Autodesk Inventor part; units mm, degrees
(part 2 of 2)
  line L254 (8.0901, 0.2026) -> (9.8203, 0.2026)
  line L255 (9.8203, 0.2026) -> (9.8203, -0.2399)
  spline S290 degree 2 poles (9.5423, 2.2873) (9.582, 2.2334) (9.7239, 2.0519) (9.7664, 1.9668) knots 0 0 0 1 2 2 2
  spline S291 degree 2 poles (9.7664, 1.9668) (9.8288, 1.8505) (9.894, 1.6321) (9.894, 1.4335) knots 0 0 0 1 2 2 2
  spline S292 degree 2 poles (9.894, 1.4335) (9.894, 1.2719) (9.7721, 0.9797) (9.6615, 0.8691) knots 0 0 0 1 2 2 2
  spline S293 degree 2 poles (9.6615, 0.8691) (9.5537, 0.7642) (9.236, 0.6365) (9.0602, 0.6365) knots 0 0 0 1 2 2 2
  spline S294 degree 2 poles (9.0602, 0.6365) (8.7879, 0.6365) (8.4021, 0.8663) (8.2915, 1.1159) knots 0 0 0 1 2 2 2
  spline S295 degree 2 poles (8.2915, 1.1159) (8.1894, 1.3371) (8.1128, 1.9384) (8.093, 2.2873) knots 0 0 0 1 2 2 2
  line L256 (8.093, 2.2873) -> (8.0079, 2.2873)
  spline S296 degree 2 poles (8.0079, 2.2873) (7.8547, 2.2873) (7.6647, 2.1937) (7.6108, 2.1086) knots 0 0 0 1 2 2 2
  spline S297 degree 2 poles (7.6108, 2.1086) (7.5569, 2.0235) (7.5229, 1.7796) (7.5229, 1.6491) knots 0 0 0 1 2 2 2
  spline S298 degree 2 poles (7.5229, 1.6491) (7.5229, 1.4959) (7.6136, 1.0818) (7.7016, 0.8748) knots 0 0 0 1 2 2 2
  line L257 (7.7016, 0.8748) -> (7.7016, 0.8493)
  line L258 (7.7016, 0.8493) -> (7.2506, 0.8493)
  spline S299 degree 2 poles (7.2506, 0.8493) (7.2166, 0.9712) (7.1315, 1.4279) (7.1315, 1.6519) knots 0 0 0 1 2 2 2
  spline S300 degree 2 poles (7.1315, 1.6519) (7.1315, 1.9242) (7.2166, 2.2958) (7.3272, 2.4433) knots 0 0 0 1 2 2 2
  spline S301 degree 2 poles (7.3272, 2.4433) (7.435, 2.5879) (7.7781, 2.7297) (8.0249, 2.7297) knots 0 0 0 1 2 2 2
  line L259 (8.0249, 2.7297) -> (9.8203, 2.7297)
  line L260 (9.8203, 2.7297) -> (9.8203, 2.2873)
  line L261 (9.8203, 2.2873) -> (9.5423, 2.2873)
  line L262 (9.1736, 2.2873) -> (8.4447, 2.2873)
  spline S302 degree 2 poles (8.4447, 2.2873) (8.4589, 2.1284) (8.5071, 1.6491) (8.5525, 1.4988) knots 0 0 0 1 2 2 2
  spline S303 degree 2 poles (8.5525, 1.4988) (8.6063, 1.3229) (8.8304, 1.0932) (9.029, 1.0932) knots 0 0 0 1 2 2 2
  spline S304 degree 2 poles (9.029, 1.0932) (9.2559, 1.0932) (9.4856, 1.3484) (9.4856, 1.5924) knots 0 0 0 1 2 2 2
  spline S305 degree 2 poles (9.4856, 1.5924) (9.4856, 1.7994) (9.3069, 2.1398) (9.1736, 2.2873) knots 0 0 0 1 2 2 2
  line L263 (9.8203, 5.3703) -> (9.8203, 4.9279)
  line L264 (9.8203, 4.9279) -> (9.5537, 4.9279)
  spline S306 degree 2 poles (9.5537, 4.9279) (9.6388, 4.8258) (9.7522, 4.6754) (9.8004, 4.5733) knots 0 0 0 1 2 2 2
  spline S307 degree 2 poles (9.8004, 4.5733) (9.8458, 4.4797) (9.894, 4.2784) (9.894, 4.145) knots 0 0 0 1 2 2 2
  spline S308 degree 2 poles (9.894, 4.145) (9.894, 3.9295) (9.7153, 3.5664) (9.5423, 3.4388) knots 0 0 0 1 2 2 2
  spline S309 degree 2 poles (9.5423, 3.4388) (9.3693, 3.3112) (8.8588, 3.1694) (8.5269, 3.1694) knots 0 0 0 1 2 2 2
  spline S310 degree 2 poles (8.5269, 3.1694) (8.1809, 3.1694) (7.676, 3.348) (7.486, 3.504) knots 0 0 0 1 2 2 2
  spline S311 degree 2 poles (7.486, 3.504) (7.3158, 3.6487) (7.1201, 4.0543) (7.1201, 4.2784) knots 0 0 0 1 2 2 2
  spline S312 degree 2 poles (7.1201, 4.2784) (7.1201, 4.4741) (7.208, 4.7662) (7.2988, 4.9279) knots 0 0 0 1 2 2 2
  line L265 (7.2988, 4.9279) -> (6.1643, 4.9279)
  line L266 (6.1643, 4.9279) -> (6.1643, 5.3703)
  line L267 (6.1643, 5.3703) -> (9.8203, 5.3703)
  line L268 (9.1821, 4.9279) -> (7.6647, 4.9279)
  spline S313 degree 2 poles (7.6647, 4.9279) (7.5853, 4.7634) (7.5257, 4.5024) (7.5257, 4.3521) knots 0 0 0 1 2 2 2
  spline S314 degree 2 poles (7.5257, 4.3521) (7.5257, 4.0117) (8.0362, 3.626) (8.5184, 3.626) knots 0 0 0 1 2 2 2
  spline S315 degree 2 poles (8.5184, 3.626) (8.9836, 3.626) (9.4743, 3.921) (9.4743, 4.2472) knots 0 0 0 1 2 2 2
  spline S316 degree 2 poles (9.4743, 4.2472) (9.4743, 4.4202) (9.3154, 4.7719) (9.1821, 4.9279) knots 0 0 0 1 2 2 2
  spline S317 degree 2 poles (9.8827, 8.5243) (9.8827, 8.1442) (9.7239, 7.611) (9.6104, 7.3756) knots 0 0 0 1 2 2 2
  line L269 (9.6104, 7.3756) -> (9.0261, 7.3756)
  line L270 (9.0261, 7.3756) -> (9.0261, 7.4096)
  spline S318 degree 2 poles (9.0261, 7.4096) (9.2417, 7.6394) (9.4799, 8.2208) (9.4799, 8.4903) knots 0 0 0 1 2 2 2
  spline S319 degree 2 poles (9.4799, 8.4903) (9.4799, 8.876) (9.1594, 9.2702) (8.8956, 9.2702) knots 0 0 0 1 2 2 2
  spline S320 degree 2 poles (8.8956, 9.2702) (8.6858, 9.2702) (8.4248, 9.0632) (8.3596, 8.8391) knots 0 0 0 1 2 2 2
  spline S321 degree 2 poles (8.3596, 8.8391) (8.3142, 8.6775) (8.2518, 8.408) (8.2008, 8.2066) knots 0 0 0 1 2 2 2
  spline S322 degree 2 poles (8.2008, 8.2066) (8.1525, 8.0251) (8.0079, 7.7386) (7.8916, 7.628) knots 0 0 0 1 2 2 2
  spline S323 degree 2 poles (7.8916, 7.628) (7.7753, 7.5202) (7.4633, 7.4011) (7.2591, 7.4011) knots 0 0 0 1 2 2 2
  spline S324 degree 2 poles (7.2591, 7.4011) (6.8337, 7.4011) (6.2579, 8.0648) (6.2579, 8.5782) knots 0 0 0 1 2 2 2
  spline S325 degree 2 poles (6.2579, 8.5782) (6.2579, 8.8732) (6.3742, 9.395) (6.4848, 9.6191) knots 0 0 0 1 2 2 2
  line L271 (6.4848, 9.6191) -> (7.0407, 9.6191)
  line L272 (7.0407, 9.6191) -> (7.0407, 9.5851)
  spline S326 degree 2 poles (7.0407, 9.5851) (6.8875, 9.4177) (6.6606, 8.8959) (6.6606, 8.6094) knots 0 0 0 1 2 2 2
  spline S327 degree 2 poles (6.6606, 8.6094) (6.6606, 8.286) (6.9641, 7.8861) (7.2109, 7.8861) knots 0 0 0 1 2 2 2
  spline S328 degree 2 poles (7.2109, 7.8861) (7.4321, 7.8861) (7.6959, 8.1215) (7.7555, 8.3428) knots 0 0 0 1 2 2 2
  spline S329 degree 2 poles (7.7555, 8.3428) (7.7952, 8.4903) (7.8973, 8.9185) (7.9398, 9.0604) knots 0 0 0 1 2 2 2
  spline S330 degree 2 poles (7.9398, 9.0604) (8.0504, 9.4206) (8.4957, 9.7553) (8.8219, 9.7553) knots 0 0 0 1 2 2 2
  spline S331 degree 2 poles (8.8219, 9.7553) (9.029, 9.7553) (9.426, 9.5879) (9.565, 9.4376) knots 0 0 0 1 2 2 2
  spline S332 degree 2 poles (9.565, 9.4376) (9.7182, 9.2702) (9.8827, 8.8448) (9.8827, 8.5243) knots 0 0 0 1 2 2 2
  spline S333 degree 2 poles (9.5423, 11.6584) (9.582, 11.6045) (9.7239, 11.423) (9.7664, 11.3379) knots 0 0 0 1 2 2 2
  spline S334 degree 2 poles (9.7664, 11.3379) (9.8288, 11.2216) (9.894, 11.0032) (9.894, 10.8047) knots 0 0 0 1 2 2 2
  spline S335 degree 2 poles (9.894, 10.8047) (9.894, 10.643) (9.7721, 10.3509) (9.6615, 10.2403) knots 0 0 0 1 2 2 2
  spline S336 degree 2 poles (9.6615, 10.2403) (9.5537, 10.1353) (9.236, 10.0077) (9.0602, 10.0077) knots 0 0 0 1 2 2 2
  spline S337 degree 2 poles (9.0602, 10.0077) (8.7879, 10.0077) (8.4021, 10.2374) (8.2915, 10.487) knots 0 0 0 1 2 2 2
  spline S338 degree 2 poles (8.2915, 10.487) (8.1894, 10.7083) (8.1128, 11.3096) (8.093, 11.6584) knots 0 0 0 1 2 2 2
  line L273 (8.093, 11.6584) -> (8.0079, 11.6584)
  spline S339 degree 2 poles (8.0079, 11.6584) (7.8547, 11.6584) (7.6647, 11.5648) (7.6108, 11.4797) knots 0 0 0 1 2 2 2
  spline S340 degree 2 poles (7.6108, 11.4797) (7.5569, 11.3946) (7.5229, 11.1507) (7.5229, 11.0202) knots 0 0 0 1 2 2 2
  spline S341 degree 2 poles (7.5229, 11.0202) (7.5229, 10.8671) (7.6136, 10.453) (7.7016, 10.2459) knots 0 0 0 1 2 2 2
  line L274 (7.7016, 10.2459) -> (7.7016, 10.2204)
  line L275 (7.7016, 10.2204) -> (7.2506, 10.2204)
  spline S342 degree 2 poles (7.2506, 10.2204) (7.2166, 10.3424) (7.1315, 10.799) (7.1315, 11.0231) knots 0 0 0 1 2 2 2
  spline S343 degree 2 poles (7.1315, 11.0231) (7.1315, 11.2954) (7.2166, 11.6669) (7.3272, 11.8144) knots 0 0 0 1 2 2 2
  spline S344 degree 2 poles (7.3272, 11.8144) (7.435, 11.9591) (7.7781, 12.1009) (8.0249, 12.1009) knots 0 0 0 1 2 2 2
  line L276 (8.0249, 12.1009) -> (9.8203, 12.1009)
  line L277 (9.8203, 12.1009) -> (9.8203, 11.6584)
  line L278 (9.8203, 11.6584) -> (9.5423, 11.6584)
  line L279 (9.1736, 11.6584) -> (8.4447, 11.6584)
  spline S345 degree 2 poles (8.4447, 11.6584) (8.4589, 11.4996) (8.5071, 11.0202) (8.5525, 10.8699) knots 0 0 0 1 2 2 2
  spline S346 degree 2 poles (8.5525, 10.8699) (8.6063, 10.6941) (8.8304, 10.4643) (9.029, 10.4643) knots 0 0 0 1 2 2 2
  spline S347 degree 2 poles (9.029, 10.4643) (9.2559, 10.4643) (9.4856, 10.7196) (9.4856, 10.9635) knots 0 0 0 1 2 2 2
  spline S348 degree 2 poles (9.4856, 10.9635) (9.4856, 11.1706) (9.3069, 11.5109) (9.1736, 11.6584) knots 0 0 0 1 2 2 2
  line L280 (9.8203, 13.173) -> (9.8203, 12.7305)
  line L281 (9.8203, 12.7305) -> (7.1939, 12.7305)
  line L282 (7.1939, 12.7305) -> (7.1939, 13.173)
  line L283 (7.1939, 13.173) -> (9.8203, 13.173)
  line L284 (6.7571, 13.2042) -> (6.7571, 12.7022)
  line L285 (6.7571, 12.7022) -> (6.2976, 12.7022)
  line L286 (6.2976, 12.7022) -> (6.2976, 13.2042)
  line L287 (6.2976, 13.2042) -> (6.7571, 13.2042)
  line L288 (6.5897, 15.2038) -> (6.5897, 15.1811)
  spline S349 degree 2 poles (6.5897, 15.1811) (6.567, 15.1215) (6.5273, 14.9003) (6.5273, 14.8124) knots 0 0 0 1 2 2 2
  spline S350 degree 2 poles (6.5273, 14.8124) (6.5273, 14.5344) (6.7769, 14.2962) (7.1059, 14.2962) knots 0 0 0 1 2 2 2
  line L289 (7.1059, 14.2962) -> (7.1939, 14.2962)
  line L290 (7.1939, 14.2962) -> (7.1939, 15.0279)
  line L291 (7.1939, 15.0279) -> (7.5598, 15.0279)
  line L292 (7.5598, 15.0279) -> (7.5598, 14.3104)
  line L293 (7.5598, 14.3104) -> (9.8203, 14.3104)
  line L294 (9.8203, 14.3104) -> (9.8203, 13.8679)
  line L295 (9.8203, 13.8679) -> (7.5598, 13.8679)
  line L296 (7.5598, 13.8679) -> (7.5598, 13.5701)
  line L297 (7.5598, 13.5701) -> (7.1939, 13.5701)
  line L298 (7.1939, 13.5701) -> (7.1939, 13.8679)
  line L299 (7.1939, 13.8679) -> (7.1059, 13.8679)
  spline S351 degree 2 poles (7.1059, 13.8679) (6.6351, 13.8679) (6.1416, 14.3245) (6.1416, 14.75) knots 0 0 0 1 2 2 2
  spline S352 degree 2 poles (6.1416, 14.75) (6.1416, 14.8719) (6.1671, 15.1074) (6.1841, 15.2038) knots 0 0 0 1 2 2 2
  line L300 (6.1841, 15.2038) -> (6.5897, 15.2038)
  line L301 (9.8203, 17.3963) -> (9.8203, 16.9538)
  line L302 (9.8203, 16.9538) -> (9.531, 16.9538)
  spline S353 degree 2 poles (9.531, 16.9538) (9.7097, 16.7496) (9.894, 16.3837) (9.894, 16.1568) knots 0 0 0 1 2 2 2
  spline S354 degree 2 poles (9.894, 16.1568) (9.894, 15.9866) (9.7806, 15.6831) (9.6586, 15.5725) knots 0 0 0 1 2 2 2
  spline S355 degree 2 poles (9.6586, 15.5725) (9.5367, 15.4591) (9.1651, 15.3343) (8.8985, 15.3343) knots 0 0 0 1 2 2 2
  line L303 (8.8985, 15.3343) -> (7.1939, 15.3343)
  line L304 (7.1939, 15.3343) -> (7.1939, 15.7767)
  line L305 (7.1939, 15.7767) -> (8.6914, 15.7767)
  spline S356 degree 2 poles (8.6914, 15.7767) (8.9013, 15.7767) (9.1764, 15.8079) (9.2786, 15.8618) knots 0 0 0 1 2 2 2
  spline S357 degree 2 poles (9.2786, 15.8618) (9.3807, 15.9157) (9.4743, 16.1001) (9.4743, 16.2731) knots 0 0 0 1 2 2 2
  spline S358 degree 2 poles (9.4743, 16.2731) (9.4743, 16.4348) (9.2899, 16.8006) (9.1566, 16.9538) knots 0 0 0 1 2 2 2
  line L306 (9.1566, 16.9538) -> (7.1939, 16.9538)
  line L307 (7.1939, 16.9538) -> (7.1939, 17.3963)
  line L308 (7.1939, 17.3963) -> (9.8203, 17.3963)
  line L309 (9.8203, 20.0567) -> (9.8203, 19.6143)
  line L310 (9.8203, 19.6143) -> (9.5537, 19.6143)
  spline S359 degree 2 poles (9.5537, 19.6143) (9.6388, 19.5121) (9.7522, 19.3618) (9.8004, 19.2597) knots 0 0 0 1 2 2 2
  spline S360 degree 2 poles (9.8004, 19.2597) (9.8458, 19.1661) (9.894, 18.9647) (9.894, 18.8314) knots 0 0 0 1 2 2 2
  spline S361 degree 2 poles (9.894, 18.8314) (9.894, 18.6159) (9.7153, 18.2528) (9.5423, 18.1252) knots 0 0 0 1 2 2 2
  spline S362 degree 2 poles (9.5423, 18.1252) (9.3693, 17.9976) (8.8588, 17.8557) (8.5269, 17.8557) knots 0 0 0 1 2 2 2
  spline S363 degree 2 poles (8.5269, 17.8557) (8.1809, 17.8557) (7.676, 18.0344) (7.486, 18.1904) knots 0 0 0 1 2 2 2
  spline S364 degree 2 poles (7.486, 18.1904) (7.3158, 18.3351) (7.1201, 18.7407) (7.1201, 18.9647) knots 0 0 0 1 2 2 2
  spline S365 degree 2 poles (7.1201, 18.9647) (7.1201, 19.1604) (7.208, 19.4526) (7.2988, 19.6143) knots 0 0 0 1 2 2 2
  line L311 (7.2988, 19.6143) -> (6.1643, 19.6143)
  line L312 (6.1643, 19.6143) -> (6.1643, 20.0567)
  line L313 (6.1643, 20.0567) -> (9.8203, 20.0567)
  line L314 (9.1821, 19.6143) -> (7.6647, 19.6143)
  spline S366 degree 2 poles (7.6647, 19.6143) (7.5853, 19.4497) (7.5257, 19.1888) (7.5257, 19.0385) knots 0 0 0 1 2 2 2
  spline S367 degree 2 poles (7.5257, 19.0385) (7.5257, 18.6981) (8.0362, 18.3124) (8.5184, 18.3124) knots 0 0 0 1 2 2 2
  spline S368 degree 2 poles (8.5184, 18.3124) (8.9836, 18.3124) (9.4743, 18.6074) (9.4743, 18.9335) knots 0 0 0 1 2 2 2
  spline S369 degree 2 poles (9.4743, 18.9335) (9.4743, 19.1066) (9.3154, 19.4583) (9.1821, 19.6143) knots 0 0 0 1 2 2 2
  line L315 (9.8203, 22.7172) -> (9.8203, 22.2747)
  line L316 (9.8203, 22.2747) -> (9.5537, 22.2747)
  spline S370 degree 2 poles (9.5537, 22.2747) (9.6388, 22.1726) (9.7522, 22.0223) (9.8004, 21.9202) knots 0 0 0 1 2 2 2
  spline S371 degree 2 poles (9.8004, 21.9202) (9.8458, 21.8266) (9.894, 21.6252) (9.894, 21.4919) knots 0 0 0 1 2 2 2
  spline S372 degree 2 poles (9.894, 21.4919) (9.894, 21.2763) (9.7153, 20.9133) (9.5423, 20.7856) knots 0 0 0 1 2 2 2
  spline S373 degree 2 poles (9.5423, 20.7856) (9.3693, 20.658) (8.8588, 20.5162) (8.5269, 20.5162) knots 0 0 0 1 2 2 2
  spline S374 degree 2 poles (8.5269, 20.5162) (8.1809, 20.5162) (7.676, 20.6949) (7.486, 20.8509) knots 0 0 0 1 2 2 2
  spline S375 degree 2 poles (7.486, 20.8509) (7.3158, 20.9955) (7.1201, 21.4011) (7.1201, 21.6252) knots 0 0 0 1 2 2 2
  spline S376 degree 2 poles (7.1201, 21.6252) (7.1201, 21.8209) (7.208, 22.113) (7.2988, 22.2747) knots 0 0 0 1 2 2 2
  line L317 (7.2988, 22.2747) -> (6.1643, 22.2747)
  line L318 (6.1643, 22.2747) -> (6.1643, 22.7172)
  line L319 (6.1643, 22.7172) -> (9.8203, 22.7172)
  line L320 (9.1821, 22.2747) -> (7.6647, 22.2747)
  spline S377 degree 2 poles (7.6647, 22.2747) (7.5853, 22.1102) (7.5257, 21.8493) (7.5257, 21.6989) knots 0 0 0 1 2 2 2
  spline S378 degree 2 poles (7.5257, 21.6989) (7.5257, 21.3586) (8.0362, 20.9728) (8.5184, 20.9728) knots 0 0 0 1 2 2 2
  spline S379 degree 2 poles (8.5184, 20.9728) (8.9836, 20.9728) (9.4743, 21.2678) (9.4743, 21.594) knots 0 0 0 1 2 2 2
  spline S380 degree 2 poles (9.4743, 21.594) (9.4743, 21.767) (9.3154, 22.1187) (9.1821, 22.2747) knots 0 0 0 1 2 2 2
  line L321 (9.8203, 23.8091) -> (9.8203, 23.3667)
  line L322 (9.8203, 23.3667) -> (7.1939, 23.3667)
  line L323 (7.1939, 23.3667) -> (7.1939, 23.8091)
  line L324 (7.1939, 23.8091) -> (9.8203, 23.8091)
  line L325 (6.7571, 23.8403) -> (6.7571, 23.3383)
  line L326 (6.7571, 23.3383) -> (6.2976, 23.3383)
  line L327 (6.2976, 23.3383) -> (6.2976, 23.8403)
  line L328 (6.2976, 23.8403) -> (6.7571, 23.8403)
  line L329 (9.8203, 26.5207) -> (9.8203, 26.0782)
  line L330 (9.8203, 26.0782) -> (8.3227, 26.0782)
  spline S381 degree 2 poles (8.3227, 26.0782) (8.1412, 26.0782) (7.8292, 26.0442) (7.7356, 25.9931) knots 0 0 0 1 2 2 2
  spline S382 degree 2 poles (7.7356, 25.9931) (7.6363, 25.9392) (7.5399, 25.7463) (7.5399, 25.5818) knots 0 0 0 1 2 2 2
  spline S383 degree 2 poles (7.5399, 25.5818) (7.5399, 25.4173) (7.7157, 25.0685) (7.8576, 24.9011) knots 0 0 0 1 2 2 2
  line L331 (7.8576, 24.9011) -> (9.8203, 24.9011)
  line L332 (9.8203, 24.9011) -> (9.8203, 24.4587)
  line L333 (9.8203, 24.4587) -> (7.1939, 24.4587)
  line L334 (7.1939, 24.4587) -> (7.1939, 24.9011)
  line L335 (7.1939, 24.9011) -> (7.486, 24.9011)
  spline S384 degree 2 poles (7.486, 24.9011) (7.3073, 25.0997) (7.1201, 25.4826) (7.1201, 25.6981) knots 0 0 0 1 2 2 2
  spline S385 degree 2 poles (7.1201, 25.6981) (7.1201, 26.0839) (7.6307, 26.5207) (8.1157, 26.5207) knots 0 0 0 1 2 2 2
  line L336 (8.1157, 26.5207) -> (9.8203, 26.5207)
  constraints: 2 end point, 1 horizontal, 1 midpoint, 2 other
extrude "Extrusion2" cut sketch "Sketch3" against normal blind 1
body "Solid1"
